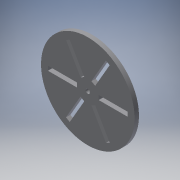
# Autodesk Inventor part: Барабан
Saved by Autodesk Inventor 2019 (Build 230136000, 136)
## iProperties
Created: 2022-06-28
Part Number: Барабан
Material: Типовые
Document SubType Name: Modeling
Designer: korsh
Density: 1 g/cm^3
Appearance: По умолчанию
Author: korsh
Autodesk Inventor part; units mm, degrees
ref_plane "YZ Plane" through (0, 0, 0) normal (1, 0, 0) x (0, 1, 0)
ref_plane "XZ Plane" through (0, 0, 0) normal (0, 1, 0) x (-1, 0, 0)
ref_plane "XY Plane" through (0, 0, 0) normal (0, 0, 1) x (1, 0, 0)
sketch "Эскиз1" plane through (0, 0, 0) normal (0, 0, 1) x (1, 0, 0)
  circle A0 centre (7, 0.0001) radius 3 projected
  circle A1 centre (7, 0.0001) radius 64.5
  point P0 (0, 0)
  dimension "d0" = 129
  constraints: 1 centre point, 1 coincident
  measures "d0" diameter of A1
extrude "Выдавливание1" add sketch "Эскиз1" along normal blind 6
sketch "Эскиз2" plane through (7, 0.0001, 6) normal (0, 0, 1) x (1, 0, 0)
  circle A0 centre (0, 0) radius 3 projected
  circle A1 centre (0, 0) radius 3 projected
  line L0 (2.5, 1.6583) -> (2.5, -1.6583)
  point P0 (-7, -0.0001)
  dimension "d3" = 2.5
  constraints: 2 end point, 2 point on circle, 1 vertical
  measures "d3" distance from line of L0 A0.centre
extrude "Выдавливание2" add sketch "Эскиз2" against normal blind 6 contours A0 L0 picked at (2.5914, -0.3806)
sketch "Эскиз3" plane through (7, 0.0001, 6) normal (0, 0, 1) x (1, 0, 0)
  line L0 (55, 3) -> (15, 3)
  line L1 (15, 3) -> (15, -3)
  line L2 (15, -3) -> (55, -3)
  line L3 (55, -3) -> (55, 3)
  circle A0 centre (0, 0) radius 3 projected
  line L4 (24.9019, 49.1314) -> (4.9019, 14.4904)
  line L5 (4.9019, 14.4904) -> (10.0981, 11.4904)
  line L6 (10.0981, 11.4904) -> (30.0981, 46.1314)
  line L7 (30.0981, 46.1314) -> (24.9019, 49.1314)
  line L8 (-30.0981, 46.1314) -> (-10.0981, 11.4904)
  line L9 (-10.0981, 11.4904) -> (-4.9019, 14.4904)
  line L10 (-4.9019, 14.4904) -> (-24.9019, 49.1314)
  line L11 (-24.9019, 49.1314) -> (-30.0981, 46.1314)
  line L12 (-55, -3) -> (-15, -3)
  line L13 (-15, -3) -> (-15, 3)
  line L14 (-15, 3) -> (-55, 3)
  line L15 (-55, 3) -> (-55, -3)
  line L16 (-24.9019, -49.1314) -> (-4.9019, -14.4904)
  line L17 (-4.9019, -14.4904) -> (-10.0981, -11.4904)
  line L18 (-10.0981, -11.4904) -> (-30.0981, -46.1314)
  line L19 (-30.0981, -46.1314) -> (-24.9019, -49.1314)
  line L20 (30.0981, -46.1314) -> (10.0981, -11.4904)
  line L21 (10.0981, -11.4904) -> (4.9019, -14.4904)
  line L22 (4.9019, -14.4904) -> (24.9019, -49.1314)
  line L23 (24.9019, -49.1314) -> (30.0981, -46.1314)
  point P0 (-7, -0.0001)
  dimension "d6" = 40
  dimension "d7" = 15
  dimension "d8" = 6
  dimension "d9" = 3
  dimension "d12" = 360
  constraints: 48 end point, 2 parallel, 1 horizontal, 1 perpendicular, 49 other
  measures "d6" distance of L1.end L2.end
  measures "d7" distance from line of L1 A0.centre
  measures "d8" distance between parallel lines of L0 L2
  measures "d9" distance from line of A0.centre L2
extrude "Выдавливание3" cut sketch "Эскиз3" against normal blind 6 contours L3 L2 L1 L0 | L7 L6 L5 L4 | L11 L10 L9 L8 | L15 L14 L13 L12 | L19 L18 L17 L16 | L23 L22 L21 L20
